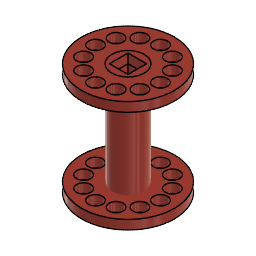
suport cifre (Autodesk Fusion 360 design; units mm, degrees)
part number: 2026-05-04-02-16-29-331
Autodesk Fusion 360 part; units mm, degrees
sketch "Sketch1" plane through (0, 0, 0) normal (0, 0, 1) x (1, 0, 0)
  circle A0 centre (0, 0) radius 10
  circle A1 centre (7, 0) radius 1.5
  circle A2 centre (0, 0) radius 3.5
  line L0 (0, 0) -> (-2, 0)
  line L1 (-2, 0) -> (-2, -2)
  line L2 (-2, -2) -> (2, -2)
  line L3 (2, -2) -> (2, 2)
  line L4 (2, 2) -> (-2, 2)
  line L5 (-2, 2) -> (-2, 0)
  dimension "d3" = 20
  dimension "d4" = 3
  dimension "d11" = 7
  dimension "d14" = 7
  dimension "d22" = 2
  dimension "d23" = 2
  dimension "d24" = 4
  dimension "d25" = 4
  dimension "d26" = 4
  constraint coincident A0.centre A2.centre
  constraint horizontal L0
  constraint perpendicular L0 L1
  constraint perpendicular L1 L2
  constraint perpendicular L0 L3
  constraint perpendicular L3 L4
  measures "d3" diameter of A0
  measures "d4" diameter of A1
  measures "d11" diameter of A2
  measures "d14" distance of A0.centre A1.centre
  measures "d22" distance of A0.centre L0.end
  measures "d23" distance of L0.end L1.end
  measures "d24" distance of L1.end L2.end
  measures "d25" distance of L2.end L3.end
  measures "d26" distance of L3.end L4.end
extrude "Extrude1" add sketch "Sketch1" along normal blind 2 contours A0 | A1 | A2 | L1 L2 L3 L4 L5 makes body 1
extrude "Extrude2" cut sketch "Sketch1" along normal blind 2 contours A1 bodies 1
pattern_circular "C-Pattern1" count 12 over 360 about axis through (0, 0, 1.75) along (0, 0, 1) of "Extrude2"
extrude "Extrude3" add sketch "Sketch1" along normal blind 24 separate body contours A2 | L1 L2 L3 L4 L5 makes body 2
copy_body "CopyPasteBodies1" bodies 1 makes body 3
move_body "Move1" bodies 3 to x (1, 0, 0) y (0, 1, 0) z (0, 0, 1) at (0, 0, 22)
extrude "Extrude5" cut sketch "Sketch1" along normal blind 90 contours L1 L2 L3 L4 L5 bodies 1 2 3
equation "d23 = d22"
equation "d24 = d22 * 2"
equation "d25 = d22 * 2"
equation "d26 = d22 * 2"
